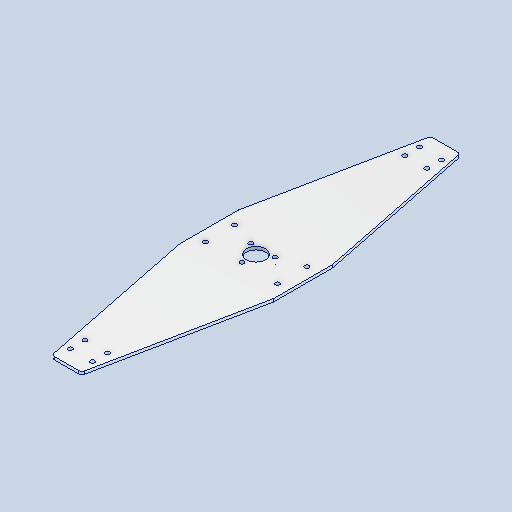
# Autodesk Inventor part: hand-grab-v2-Plate-m=F
Saved by Autodesk Inventor 2025.1 (Build 291241000, 241)
## iProperties
Created: 2024-10-12
Part Number: hand-grab-v2-Plate-m=F
Material: アルミニウム 6061
Document SubType Name: Modeling
Designer: haruy
Density: 2.7 g/cm^3
Appearance: アルミニウム - フラット
Author: haruy
Autodesk Inventor part; units mm, degrees
ref_plane "YZ Plane" through (0, 0, 0) normal (1, 0, 0) x (0, 1, 0)
ref_plane "XZ Plane" through (0, 0, 0) normal (0, 1, 0) x (-1, 0, 0)
ref_plane "XY Plane" through (0, 0, 0) normal (0, 0, 1) x (1, 0, 0)
derived "hand-grab-v2-Sketch-Base.ipt"
sketch "スケッチ1" plane through (300, 0, 0) normal (1, 0, 0) x (0, 1, 0)
  circle A0 centre (0, 0) radius 122.5
  line L0 (-136.5, 142.5) -> (-132.5, 142.5)
  line L1 (-132.5, 142.5) -> (-132.5, -206.7109)
  line L2 (-132.5, -206.7109) -> (-136.5, -206.7109)
  line L3 (-136.5, -206.7109) -> (-136.5, 142.5)
  line L4 (0, 0) -> (86.6206, 86.6206)
  line L5 (0, 0) -> (0, 122.5)
  line L6 (0, 0) -> (-61.25, 106.0881)
  line L7 (-150.5, 12.2) -> (-198.3, 12.2)
  line L8 (-198.3, 12.2) -> (-198.3, -12.2)
  line L9 (-198.3, -12.2) -> (-150.5, -12.2)
  line L10 (-150.5, -12.2) -> (-150.5, 12.2)
  line L11 (-150.5, 6.5) -> (-147.9, 6.5)
  line L12 (-147.9, 6.5) -> (-147.9, -6.5)
  line L13 (-147.9, -6.5) -> (-150.5, -6.5)
  line L14 (-150.5, -6.5) -> (-150.5, 6.5)
  line L15 (-147.9, 3) -> (-133.5, 3)
  line L16 (-133.5, 3) -> (-133.5, -3)
  line L17 (-133.5, -3) -> (-147.9, -3)
  line L18 (-147.9, -3) -> (-147.9, 3)
  line L19 (-146.5, 70.3296) -> (-150.5, 70.3296)
  line L20 (-150.5, 70.3296) -> (-150.5, -72.1331)
  line L21 (-150.5, -72.1331) -> (-146.5, -72.1331)
  line L22 (-146.5, -72.1331) -> (-146.5, 70.3296)
  line L23 (-136.5, 9) -> (-142.5, 9)
  line L24 (-142.5, 9) -> (-142.5, -9)
  line L25 (-142.5, -9) -> (-136.5, -9)
  line L26 (-136.5, -9) -> (-136.5, 9)
  line L27 (-61.25, 106.0881) -> (-132.5, 106.0881)
  circle A1 centre (-532.5, 0) radius 600
  line L28 (-132.5, 142.5) -> (-7.6064, 142.5)
  arc A2 (86.6206, 86.6206) -> (-7.6064, 142.5) centre (3, 53) ccw
  circle A3 centre (-532.5, 0) radius 400
  circle A4 centre (-332.5, 0) radius 600
sketch "スケッチ2" plane through (0, -300, 0) normal (0, 1, 0) x (-1, 0, 0)
  circle A0 centre (0, 0) radius 122.5 construction
  line L0 (-34, 142.5) -> (-30, 142.5)
  line L1 (-30, 142.5) -> (-30, 106) construction
  line L2 (-30, 106) -> (-34, 106) construction
  line L3 (-34, 106) -> (-34, 142.5)
  line L4 (30, 142.5) -> (34, 142.5)
  line L5 (34, 142.5) -> (34, 106)
  line L6 (34, 106) -> (30, 106)
  line L7 (30, 106) -> (30, 142.5)
  circle A1 centre (0, 0) radius 12.5
  line L8 (-30, 142.5) -> (30, 142.5)
  line L9 (-12.5, 103.9737) -> (-12.5, -60) construction
  line L10 (-12.5, -60) -> (-30, -60)
  line L11 (-30, -60) -> (-30, 142.5) construction
  line L12 (-30, 142.5) -> (-12.5, 142.5)
  line L13 (-12.5, 142.5) -> (-12.5, -60) construction
  line L14 (-30, 20) -> (-12.5, 20) construction
  line L15 (-4.5, 136) -> (4.5, 136)
  line L16 (4.5, 136) -> (4.5, 41) construction
  line L17 (4.5, 41) -> (-4.5, 41)
  line L18 (-4.5, 41) -> (-4.5, 136) construction
  line L19 (10, 128.5) -> (-10, 128.5)
  line L20 (-10, 128.5) -> (-10, 98.5)
  line L21 (-10, 98.5) -> (10, 98.5)
  line L22 (10, 98.5) -> (10, 128.5)
  line L23 (-12.5, 20) -> (-11.5, 20)
  line L24 (-11.5, 20) -> (-11.5, -60) construction
  line L25 (-11.5, -60) -> (-12.5, -60)
  line L26 (-12.5, -60) -> (-12.5, 20) construction
  line L27 (-11.5, 20) -> (-13.8, 19.214) construction
  line L28 (-13.8, 19.214) -> (-13.8, 18.429)
  line L29 (-13.8, 18.429) -> (-11.5, 17.643) construction
  line L30 (-11.5, 17.643) -> (-11.5, 20) construction
  line L31 (-11.5, 16.8584) -> (-13.8, 16.0724) construction
  line L32 (-13.8, 15.2874) -> (-11.5, 14.5014) construction
  line L33 (-13.8, 16.0724) -> (-13.8, 15.2874)
  line L34 (-11.5, 13.7168) -> (-13.8, 12.9308) construction
  line L35 (-13.8, 12.1458) -> (-11.5, 11.3598) construction
  line L36 (-13.8, 12.9308) -> (-13.8, 12.1458)
  line L37 (-11.5, 10.5752) -> (-13.8, 9.7892) construction
  line L38 (-13.8, 9.0042) -> (-11.5, 8.2182) construction
  line L39 (-13.8, 9.7892) -> (-13.8, 9.0042)
  line L40 (-11.5, 7.4336) -> (-13.8, 6.6476) construction
  line L41 (-13.8, 5.8626) -> (-11.5, 5.0766)
  line L42 (-13.8, 6.6476) -> (-13.8, 5.8626)
  line L43 (-11.5, 4.292) -> (-13.8, 3.506) construction
  line L44 (-13.8, 2.721) -> (-11.5, 1.935)
  line L45 (-13.8, 3.506) -> (-13.8, 2.721)
  line L46 (-11.5, 1.1505) -> (-13.8, 0.3645) construction
  line L47 (-13.8, -0.4205) -> (-11.5, -1.2065)
  line L48 (-13.8, 0.3645) -> (-13.8, -0.4205)
  line L49 (-11.5, -1.9911) -> (-13.8, -2.7771) construction
  line L50 (-13.8, -3.5621) -> (-11.5, -4.3481)
  line L51 (-13.8, -2.7771) -> (-13.8, -3.5621)
  line L52 (-11.5, -5.1327) -> (-13.8, -5.9187) construction
  line L53 (-13.8, -6.7037) -> (-11.5, -7.4897)
  line L54 (-13.8, -5.9187) -> (-13.8, -6.7037)
  line L55 (-11.5, -8.2743) -> (-13.8, -9.0603) construction
  line L56 (-13.8, -9.8453) -> (-11.5, -10.6313) construction
  line L57 (-13.8, -9.0603) -> (-13.8, -9.8453)
  line L58 (-11.5, -11.4159) -> (-13.8, -12.2019) construction
  line L59 (-13.8, -12.9869) -> (-11.5, -13.7729)
  line L60 (-13.8, -12.2019) -> (-13.8, -12.9869)
  line L61 (-11.5, -14.5575) -> (-13.8, -15.3435) construction
  line L62 (-13.8, -16.1285) -> (-11.5, -16.9145)
  line L63 (-13.8, -15.3435) -> (-13.8, -16.1285)
  line L64 (-11.5, -17.6991) -> (-13.8, -18.4851) construction
  line L65 (-13.8, -19.2701) -> (-11.5, -20.0561)
  line L66 (-13.8, -18.4851) -> (-13.8, -19.2701)
  line L67 (-11.5, -20.8407) -> (-13.8, -21.6267)
  line L68 (-13.8, -22.4117) -> (-11.5, -23.1977)
  line L69 (-13.8, -21.6267) -> (-13.8, -22.4117)
  line L70 (-11.5, -23.9823) -> (-13.8, -24.7683)
  line L71 (-13.8, -25.5533) -> (-11.5, -26.3393)
  line L72 (-13.8, -24.7683) -> (-13.8, -25.5533)
  line L73 (-11.5, -27.1238) -> (-13.8, -27.9099)
  line L74 (-13.8, -28.6949) -> (-11.5, -29.4809)
  line L75 (-13.8, -27.9099) -> (-13.8, -28.6949)
  line L76 (-11.5, -30.2654) -> (-13.8, -31.0514)
  line L77 (-13.8, -31.8364) -> (-11.5, -32.6224)
  line L78 (-13.8, -31.0514) -> (-13.8, -31.8364)
  line L79 (-11.5, -33.407) -> (-13.8, -34.193)
  line L80 (-13.8, -34.978) -> (-11.5, -35.764)
  line L81 (-13.8, -34.193) -> (-13.8, -34.978)
  line L82 (-11.5, -36.5486) -> (-13.8, -37.3346)
  line L83 (-13.8, -38.1196) -> (-11.5, -38.9056)
  line L84 (-13.8, -37.3346) -> (-13.8, -38.1196)
  line L85 (-11.5, -39.6902) -> (-13.8, -40.4762)
  line L86 (-13.8, -41.2612) -> (-11.5, -42.0472)
  line L87 (-13.8, -40.4762) -> (-13.8, -41.2612)
  line L88 (-11.5, -42.8318) -> (-13.8, -43.6178)
  line L89 (-13.8, -44.4028) -> (-11.5, -45.1888)
  line L90 (-13.8, -43.6178) -> (-13.8, -44.4028)
  line L91 (-11.5, -45.9734) -> (-13.8, -46.7594)
  line L92 (-13.8, -47.5444) -> (-11.5, -48.3304)
  line L93 (-13.8, -46.7594) -> (-13.8, -47.5444)
  line L94 (-11.5, -49.115) -> (-13.8, -49.901)
  line L95 (-13.8, -50.686) -> (-11.5, -51.472)
  line L96 (-13.8, -49.901) -> (-13.8, -50.686)
  line L97 (-11.5, -52.2566) -> (-13.8, -53.0426)
  line L98 (-13.8, -53.8276) -> (-11.5, -54.6136)
  line L99 (-13.8, -53.0426) -> (-13.8, -53.8276)
  line L100 (-11.5, -55.3982) -> (-13.8, -56.1842)
  line L101 (-13.8, -56.9692) -> (-11.5, -57.7552)
  line L102 (-13.8, -56.1842) -> (-13.8, -56.9692)
  line L103 (-11.5, -58.5397) -> (-13.8, -59.3258)
  line L104 (-13.8, -60.1108) -> (-11.5, -60.8968)
  line L105 (-13.8, -59.3258) -> (-13.8, -60.1108)
  line L106 (-13.8, 20) -> (-13.8, -60) construction
  line L107 (-13.8, -59.3258) -> (-30, -59.3258)
  line L108 (-13.8, 18.429) -> (-30, 18.429)
  line L109 (-13.8, 18.429) -> (-13.8, 142.5) construction
  line L110 (-34, 137.5) -> (34, 137.5)
  line L111 (-34, 117.5) -> (34, 117.5) construction
  line L112 (30, 106) -> (-13.8, 106)
  line L113 (32, -142.5) -> (30, -142.5)
  line L114 (30, -142.5) -> (30, -106) construction
  line L115 (30, -106) -> (32, -106)
  line L116 (32, -106) -> (32, -142.5)
  line L117 (-32, -106) -> (-30, -106)
  line L118 (-30, -106) -> (-30, -142.5)
  line L119 (-30, -142.5) -> (-32, -142.5)
  line L120 (-32, -142.5) -> (-32, -106)
  line L121 (30, -142.5) -> (-30, -142.5)
  line L122 (30, -142.5) -> (12.5, -142.5)
  line L123 (12.5, -142.5) -> (12.5, 80) construction
  line L124 (12.5, 80) -> (30, 80)
  line L125 (30, 80) -> (30, -142.5) construction
  line L126 (-30, -106) -> (12.5, -106)
  line L127 (-4.5, -41) -> (4.5, -41)
  line L128 (4.5, -41) -> (4.5, -136) construction
  line L129 (4.5, -136) -> (-4.5, -136)
  line L130 (-4.5, -136) -> (-4.5, -41) construction
  line L131 (-10, -98.5) -> (10, -98.5)
  line L132 (10, -98.5) -> (10, -128.5)
  line L133 (10, -128.5) -> (-10, -128.5)
  line L134 (-10, -128.5) -> (-10, -98.5)
  circle A2 centre (-7.5, 118.5) radius 1.5
  line L135 (0, 128.5) -> (0, 98.5)
  line L136 (10, 113.5) -> (-10, 113.5)
  circle A3 centre (-7.5, 108.5) radius 1.5
  circle A4 centre (7.5, 118.5) radius 1.5
  circle A5 centre (7.5, 108.5) radius 1.5
  circle A6 centre (0, 0) radius 6.5
  circle A7 centre (0, 0) radius 9.5
  circle A8 centre (0, 9.5) radius 1.5
  circle A9 centre (-8.2272, -4.75) radius 1.5
  circle A10 centre (8.2272, -4.75) radius 1.5
  circle A11 centre (-7.5, -118.5) radius 1.5
  line L137 (0, -98.5) -> (0, -128.5)
  line L138 (-10, -113.5) -> (10, -113.5)
  circle A12 centre (-7.5, -108.5) radius 1.5
  circle A13 centre (7.5, -118.5) radius 1.5
  circle A14 centre (7.5, -108.5) radius 1.5
  line L139 (10, 98.5) -> (12.496, 0.3177)
  line L140 (-12.496, 0.3177) -> (-10, 98.5)
  line L141 (-32, 202.1278) -> (-17, 202.1278)
  line L142 (-17, 202.1278) -> (-17, -209.3238) construction
  line L143 (-17, -209.3238) -> (-32, -209.3238)
  line L144 (-32, -209.3238) -> (-32, 202.1278)
  line L145 (17, 202.1278) -> (32, 202.1278)
  line L146 (32, 202.1278) -> (32, -266.5661)
  line L147 (32, -266.5661) -> (17, -266.5661)
  line L148 (17, -266.5661) -> (17, 202.1278) construction
  line L149 (4.5, 41) -> (-13.8, 41)
  line L150 (-30, 30) -> (-12.65, 30)
  line L151 (-30, 142.5) -> (-15, 142.5)
  line L152 (-15, 142.5) -> (-15, 106)
  line L153 (-15, 106) -> (-30, 106)
  line L154 (-30, 106) -> (-30, 142.5)
  line L155 (30, 142.5) -> (15, 142.5)
  line L156 (15, 142.5) -> (15, 106)
  line L157 (15, 106) -> (30, 106)
  line L158 (30, 106) -> (30, 142.5)
  line L159 (-13.8, 21.571) -> (-11.5, 20.785)
  line L160 (-11.5, 20.0004) -> (-13.8, 19.2144)
  line L161 (-13.8, 24.713) -> (-11.5, 23.927)
  line L162 (-11.5, 23.1424) -> (-13.8, 22.3564)
  line L163 (-13.8, 27.855) -> (-11.5, 27.069)
  line L164 (-11.5, 26.2844) -> (-13.8, 25.4984)
  line L165 (-13.8, 30.997) -> (-11.5, 30.211)
  line L166 (-11.5, 29.4264) -> (-13.8, 28.6404)
  line L167 (-11.5, 20.0004) -> (-11.5, 27.069)
  line L168 (-13.8, 27.855) -> (-30, 27.855)
  line L169 (0, 0) -> (-32, 0)
  line L170 (10, -98.5) -> (12.496, -0.3177)
  line L171 (-12.496, -0.3177) -> (-10, -98.5)
  circle A15 centre (-24.5, 10) radius 1.5
  circle A16 centre (24.5, 10) radius 1.5
  line L172 (17, 20) -> (32, 20)
  line L173 (-32, 20) -> (-17, 20)
  line L174 (17, 20) -> (11.9956, 20)
  line L175 (-17, 20) -> (-11.9956, 20)
  line L176 (-30, -20) -> (-12.5, -20) construction
  circle A17 centre (-24.5, -10) radius 1.5
  circle A18 centre (24.5, -10) radius 1.5
  line L177 (17, -20) -> (32, -20)
  line L178 (-32, -20) -> (-17, -20)
  line L179 (17, -20) -> (11.9956, -20)
  line L180 (-17, -20) -> (-11.9956, -20)
  line L181 (-10, 128.5) -> (-32, 20)
  line L182 (10, 128.5) -> (32, 20)
  line L183 (-32, -20) -> (-10, -128.5)
  line L184 (10, -128.5) -> (32, -20)
  point P0 (21.25, -142.5)
  point P1 (-12.4976, -0.2434)
  point P2 (-12.4819, -0.871)
  point P3 (-12.4693, -0.8753)
  point P4 (-22.5, 142.5)
  dimension "d5" = 19
  dimension "d1" = 3
  dimension "d2" = 10
  dimension "d3" = 2.5
  dimension "d4" = 13
  dimension "d6" = 3
  dimension "d9" = 360
  dimension "d11" = 3
  dimension "d12" = 2.5
  dimension "d13" = 10
  dimension "d16" = 3
  dimension "d17" = 3
  dimension "d18" = 10
  dimension "d19" = 7.5
  dimension "d20" = 10
  dimension "d21" = 7.5
  dimension "d22" = 10
  dimension "d23" = 10
  measures "d1" diameter of A2
  measures "d2" distance from line of A2.centre L19
  measures "d3" distance from line of L20 A2.centre
  measures "d4" diameter of A6
  measures "d6" diameter of A8
  measures "d11" diameter of A11
  measures "d12" distance from line of A11.centre L134
  measures "d13" distance from line of L133 A11.centre
  measures "d16" diameter of A15
  measures "d17" diameter of A16
  measures "d18" distance from line of A15.centre L169
  measures "d19" distance from line of L144 A15.centre
  measures "d20" vertical distance of A16.centre point (0, 0)
  measures "d21" distance from line of A16.centre L148
  measures "d22" distance from line of L173 A15.centre
  measures "d23" distance from line of A16.centre L172
ref_plane "作業平面1" through (0, -300, 0) normal (0, 1, 0) x (-1, 0, 0)
ref_plane "作業平面2" through (300, 0, 0) normal (1, 0, 0) x (0, 1, 0)
extrude "押し出し1" add sketch "スケッチ2" along normal blind 2 contours L173 L175 L23 L140 A1 L169 L144 | L181 L20 L140 L23 L175 L173 | L169 L48 L47 L171 L180 L178 L144 | L178 L180 L171 L67 L69 L68 L70 L72 L71 L73 L75 L74 L76 L78 L77 L79 L81 L80 L82 L84 L83 L134 L126 L183 L10 L105 L107 | L169 A1 L171 L47 L48 | L19 L135 L136 L20 | L107 L105 L10 L183 | A1 | L140 L159 L167 L23 | L23 L160 L140 | L19 L22 L136 L135 | L136 L135 L112 L20 | L182 L172 L174 L139 L22 L112 | L112 L22 L182 | L171 L50 A1 L170 L131 | L47 A1 L50 L171 | L140 L44 A1 | L167 L163 L140 L21 L139 A1 L44 L160 | L140 L162 L167 L159 | L136 L22 L112 L135 | L112 L135 L21 L20 | L22 L21 L135 L112 | L126 L134 L183 | L171 L68 L69 L67 | L140 L161 L167 L162 | L146 L177 L179 L170 A1 L139 L174 L172 | L134 L131 L137 L126 | L126 L137 L138 L134 | L134 L138 L137 L133 | L140 L164 L167 L161 | L184 L132 L170 L179 L177 | L137 L131 L132 L126 | L126 L132 L138 L137 | L137 L138 L132 L133 | L171 L71 L72 L70 | L140 L163 L167 L164 | L83 L84 L82 L171 | L171 L74 L75 L73 | L80 L81 L79 L171 | L171 L77 L78 L76 | A7 A10 A9 A8
fillet "フィレット2" radius 2 8 edges at (32, -299, 20) (10, -299, 128.5) (-10, -299, 128.5) (-32, -299, 20) (-32, -299, -20) (-10, -299, -128.5) (10, -299, -128.5) (32, -299, -20)
